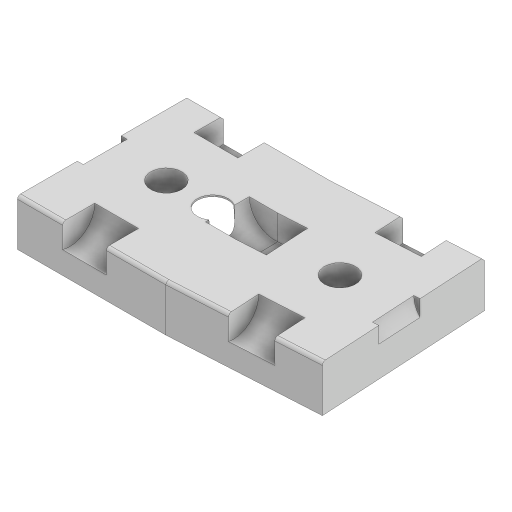
# Autodesk Inventor part: test_inventor_1
Saved by Autodesk Inventor 2024.3 (Build 283343000, 343)
## iProperties
Created: 2025-11-06
Part Number: test_inventor_1
Material: 常规
Document SubType Name: Modeling
Designer: lostcat
Density: 1 g/cm^3
Appearance: 默认
Author: lostcat
Autodesk Inventor part; units mm, degrees
ref_plane "YZ Plane" through (0, 0, 0) normal (1, 0, 0) x (0, 1, 0)
ref_plane "XZ Plane" through (0, 0, 0) normal (0, 1, 0) x (-1, 0, 0)
ref_plane "XY Plane" through (0, 0, 0) normal (0, 0, 1) x (1, 0, 0)
sketch "草图1" plane through (0, 0, 0) normal (0, 1, 0) x (-1, 0, 0)
  line L0 (-31.867922, 58.955658) -> (63.735845, 58.955658)
  line L1 (63.735845, 58.955658) -> (63.735845, -52.126817)
  line L2 (63.735845, -52.126817) -> (-28.68113, -52.126817)
  line L3 (-28.68113, -52.126817) -> (-31.867922, 58.955658)
  point P0 (0, 0)
  constraints: 8 end point, 2 perpendicular, 1 horizontal
sketch "草图1 outline for 拉伸1" plane through (0, 0, 0) normal (0, 1, 0) x (-1, 0, 0)
  line L0 (-31.867922, 58.955658) -> (-28.68113, -52.126817)
  line L1 (63.735845, 58.955658) -> (-31.867922, 58.955658)
  line L2 (63.735845, -52.126817) -> (63.735845, 58.955658)
  line L3 (-28.68113, -52.126817) -> (63.735845, -52.126817)
extrude "拉伸1" add sketch "草图1 outline for 拉伸1" along normal blind 30
sketch "草图2" plane through (0, 30, 0) normal (0, 1, 0) x (1, 0, 0)
  line L0 (27.698746, -13.010017) -> (11.471198, -13.010017)
  line L1 (11.471198, -13.010017) -> (11.471198, 15.248299)
  line L2 (11.471198, 15.248299) -> (27.698746, 15.248299)
  line L3 (27.698746, 15.248299) -> (27.698746, -13.010017)
  point P0 (0, 0)
  constraints: 8 end point, 3 perpendicular, 1 horizontal
sketch "草图2 outline for 旋转1" plane through (0, 30, 0) normal (0, 1, 0) x (1, 0, 0)
  line L0 (27.698746, -13.010017) -> (27.698746, 15.248299)
  line L1 (11.471198, -13.010017) -> (27.698746, -13.010017)
  line L2 (11.471198, 15.248299) -> (11.471198, -13.010017)
  line L3 (27.698746, 15.248299) -> (11.471198, 15.248299)
revolve "旋转1" cut sketch "草图2 outline for 旋转1" angle 360 about axis through (27.698746, 30, -15.248299) along (0, 0, 1)
fillet "圆角1" radius 2 1 edges at (-15.934, 30, 58.9557)
chamfer "倒角1" distance 2 angle 45 1 edges at (-17.5274, 30, -52.1268) measured on face at (-2.1245, 10, -52.1268)
sketch "草图3" plane through (0, 30, 0) normal (0, 1, 0) x (1, 0, 0)
  point P0 (0, 0)
  point P1 (-24.216609, -2.571345)
hole "孔1" at (-24.216609, 30, 2.571345) direction (0, -1, 0) diameter 20 end through all
pattern_circular "环形阵列1" count 4 over 360 about axis through (-24.216609, -119.597448, 2.571345) along (0, -1, 0) of "旋转1"
shell "抽壳1" thickness 1 removed faces 1 at (15.419844, 0, 3.535184)
mirror "镜像1" about plane through (31.867922, 0, 58.955658) normal (0.9995887, 0, -0.0286767)
pattern_linear "矩形阵列1" count 2 spacing 30 along (1, 0, 0) of "孔1"
